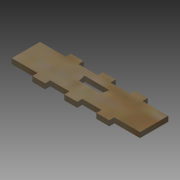
# Autodesk Inventor part: front(vga)
Saved by Autodesk Inventor 2016 (Build 200138000, 138)
## iProperties
Created: 2015-10-06
Part Number: front(vga)
Material: Generic
Document SubType Name: Modeling
Designer: Haukur
Density: 1 g/cm^3
Appearance: Plywood - Weathered
Author: Haukur
Autodesk Inventor part; units mm, degrees
ref_plane "YZ Plane" through (0, 0, 0) normal (1, 0, 0) x (0, 1, 0)
ref_plane "XZ Plane" through (0, 0, 0) normal (0, 1, 0) x (-1, 0, 0)
ref_plane "XY Plane" through (0, 0, 0) normal (0, 0, 1) x (1, 0, 0)
sketch "Sketch1" plane through (0, 0, 0) normal (0, 0, 1) x (1, 0, 0)
  line L0 (0, 4) -> (0, 26)
  line L1 (0, 26) -> (20, 26)
  line L2 (20, 26) -> (20, 30)
  line L3 (20, 30) -> (30, 30)
  line L4 (30, 30) -> (30, 26)
  line L5 (30, 26) -> (45, 26)
  line L6 (45, 26) -> (45, 30)
  line L7 (45, 30) -> (55, 30)
  line L8 (55, 30) -> (55, 26)
  line L9 (55, 26) -> (70, 26)
  line L10 (70, 26) -> (70, 30)
  line L11 (70, 30) -> (80, 30)
  line L12 (80, 30) -> (80, 26)
  line L13 (80, 26) -> (100, 26)
  line L14 (100, 26) -> (100, 4)
  line L15 (100, 4) -> (80, 4)
  line L16 (80, 4) -> (80, 0)
  line L17 (80, 0) -> (70, 0)
  line L18 (70, 0) -> (70, 4)
  line L19 (55, 4) -> (70, 4)
  line L20 (55, 4) -> (55, 0)
  line L21 (45, 0) -> (45, 4)
  line L22 (30, 4) -> (30, 0)
  line L23 (45, 4) -> (30, 4)
  line L24 (45, 0) -> (55, 0)
  line L25 (30, 0) -> (20, 0)
  line L26 (20, 4) -> (20, 0)
  line L27 (20, 4) -> (0, 4)
  point P0 (0, 0)
  dimension "d0" = 22
  dimension "d1" = 20
  dimension "d2" = 4
  dimension "d3" = 10
  dimension "d4" = 15
  dimension "d5" = 10
  dimension "d6" = 15
  dimension "d7" = 10
  dimension "d8" = 20
  dimension "d9" = 22
  dimension "d10" = 20
  constraints: 56 end point, 31 point on line, 12 perpendicular, 1 vertical
  measures "d0" distance of L0.start L0.end
  measures "d1" distance of L0.end L1.end
  measures "d2" distance of L1.end L2.end
  measures "d3" distance of L2.end L3.end
  measures "d4" distance of L4.end L5.end
  measures "d5" distance of L6.end L7.end
  measures "d6" distance of L8.end L9.end
  measures "d7" distance of L10.end L11.end
  measures "d8" distance of L12.end L13.end
  measures "d9" distance of L13.end L14.end
  measures "d10" distance of L14.end L15.end
extrude "Extrusion1" add sketch "Sketch1" along normal blind 4
sketch "Sketch2" plane through (0, 0, 4) normal (0, 0, 1) x (1, 0, 0)
  line L0 (50, 20.5) -> (40.25, 20.5)
  line L1 (40.25, 20.5) -> (59.75, 20.5)
  line L2 (50, 15) -> (58.5, 15)
  line L3 (58.5, 15) -> (41.5, 15)
  line L4 (41.5, 15) -> (40.25, 20.5)
  line L5 (58.5, 15) -> (59.75, 20.5)
  point P0 (0, 0)
  dimension "d19" = 5.5
  dimension "d20" = 9.75
  constraints: 12 end point, 2 point on line, 1 horizontal
  measures "d19" distance of L2.start L0.start
  measures "d20" distance of L0.start L0.end
extrude "Extrusion2" cut sketch "Sketch2" against normal blind 4
body "Solid1"
